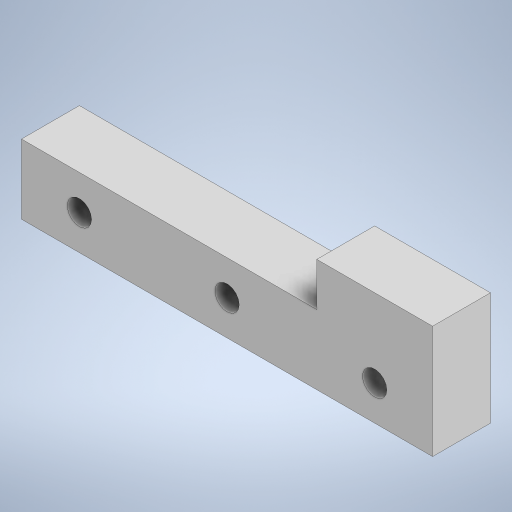
# Autodesk Inventor part: Touchscreen mount v01
Saved by Autodesk Inventor 2023 (Build 270158000, 158)
## iProperties
Created: 2024-06-28
Part Number: Touchscreen mount v01
Material: Generic
Document SubType Name: Modeling
Designer: Akramilab
Density: 1 g/cm^3
Appearance: Default
Author: Akramilab
Autodesk Inventor part; units mm, degrees
ref_plane "YZ Plane" through (0, 0, 0) normal (1, 0, 0) x (0, 1, 0)
ref_plane "XZ Plane" through (0, 0, 0) normal (0, 1, 0) x (-1, 0, 0)
ref_plane "XY Plane" through (0, 0, 0) normal (0, 0, 1) x (1, 0, 0)
sketch "Sketch1" plane through (0, 0, 0) normal (0, 0, 1) x (1, 0, 0)
  line L0 (0, 0) -> (71, 0)
  line L1 (71, 0) -> (71, -12)
  line L2 (71, -12) -> (0, -12)
  line L3 (0, -12) -> (0, 0)
  circle A0 centre (10, -6) radius 2.1
  circle A1 centre (35.5, -6) radius 2.1
  circle A2 centre (61, -6) radius 2.1
  line L4 (71, 0) -> (51, 0)
  line L5 (51, 0) -> (51, 7.5)
  line L6 (51, 7.5) -> (71, 7.5)
  line L7 (71, 7.5) -> (71, 0)
  point P0 (0, -6)
  point P1 (71, -6)
  point P2 (35.5, 0)
  dimension "d0" = 71
  dimension "d1" = 12
  dimension "d2" = 10
  dimension "d3" = 6
  dimension "d4" = 10
  dimension "d5" = 6
  dimension "d6" = 6
  dimension "d7" = 35.5
  dimension "d8" = 4.2
  dimension "d9" = 4.2
  dimension "d10" = 4.2
  dimension "d11" = 20
  dimension "d12" = 7.5
  constraints: 16 end point, 4 parallel, 3 centre point, 3 coincident, 3 midpoint, 2 horizontal, 2 perpendicular
  measures "d0" distance of L1.end L2.end
  measures "d1" distance of L0.end L1.end
  measures "d2" distance of point (10, -6) point (0, -6)
  measures "d3" distance from line of point (10, -6) L0
  measures "d4" distance of point (61, -6) point (71, -6)
  measures "d5" distance from line of point (61, -6) L2
  measures "d6" distance of point (35.5, 0) point (35.5, -6)
  measures "d7" distance from line of L3 point (35.5, -6)
  measures "d8" diameter of A0
  measures "d9" diameter of A1
  measures "d10" diameter of A2
  measures "d11" distance of L5.end L6.end
  measures "d12" distance of L4.end L5.end
extrude "Extrusion1" add sketch "Sketch1" along normal blind 10
equation "\"d3\" = 0.5 * d1"
equation "\"d4\" = d2"
equation "\"d5\" = d3"
equation "\"d6\" = d3"
equation "\"d7\" = 0.5 * d0"
equation "\"d9\" = d8"
equation "\"d10\" = d8"
body "Solid1"
